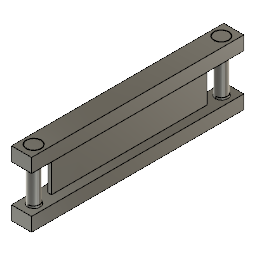
Treads v2 (Autodesk Fusion 360 design; units mm, degrees)
Autodesk Fusion 360 part; units mm, degrees
note: some values were not read from the file. Chosen so that the rebuilt part matches the saved one: which bodies a step acts on; which face or edge a step refers to.
sketch "Sketch1" plane through (0, 0, 0) normal (0, 0, 1) x (1, 0, 0)
  line L0 (0, 0) -> (11.5, 0)
  line L1 (11.5, 0) -> (11.5, 40)
  line L2 (11.5, 40) -> (0, 40)
  line L3 (0, 40) -> (0, 0)
  dimension "d1" = 11.5
  dimension "d2" = 40
  constraint horizontal L0
  constraint vertical L1
  constraint horizontal L2
  constraint vertical L3
  constraint coincident L0.start L3.end
  measures "d1" distance of L0.start L0.end
  measures "d2" distance of L0.start L2.end
extrude "Extrude1" add sketch "Sketch1" along normal blind 7.85 makes body 1
sketch "Sketch2" plane through (0, 0, 7.85) normal (0, 0, 1) x (-1, 0, 0)
  line L0 (0, -40) -> (0, 0)
  line L1 (0, 0) -> (-11.5, 0)
  line L2 (-11.5, 0) -> (-11.5, -40)
  line L3 (-11.5, -40) -> (0, -40)
  circle A0 centre (-5.6811, -7) radius 3.5
  circle A1 centre (-5.6811, -7) radius 3.25
  circle A2 centre (-5.6811, -7) radius 4
  circle A3 centre (-5.6811, -7) radius 4.25
  circle A4 centre (-5.6811, -33) radius 3.25
  circle A5 centre (-5.6811, -33) radius 3.5
  circle A6 centre (-5.6811, -33) radius 4
  circle A7 centre (-5.6811, -33) radius 4.25
  dimension "d5" = 7
  dimension "d6" = 6.5
  dimension "d7" = 8
  dimension "d12" = 8.5
  dimension "d17" = 7
  dimension "d18" = 7
  dimension "d19" = 6.5
  dimension "d20" = 8
  dimension "d21" = 8.5
  dimension "d22" = 7
  constraint concentric A0 A1
  constraint concentric A0 A2
  constraint concentric A1 A3
  constraint concentric A4 A5
  constraint concentric A5 A6
  constraint concentric A4 A7
  measures "d5" diameter of A0
  measures "d6" diameter of A1
  measures "d7" diameter of A2
  measures "d12" diameter of A3
  measures "d17" distance of L1 A0.centre
  measures "d18" diameter of A5
  measures "d19" diameter of A4
  measures "d20" diameter of A6
  measures "d21" diameter of A7
  measures "d22" distance of L3 A4.centre
extrude "Extrude2" cut sketch "Sketch2" against normal blind 2 contours A2 | A3 | A6 | A7 bodies 1
extrude "Extrude3" cut sketch "Sketch2" against normal blind 14 contours A0 | A5 bodies 1 makes body 2 at (5.8142, 1.1699, 0) makes body 3 at (2.4351, 33.162, 5.2333)
extrude "Extrude4" add sketch "Sketch2" along normal blind 1 contours A0 | A1 | A2 | A4 | A5 | A6 bodies 1 3
move_body "Move1" bodies 3 1 to x (1, 0, 0) y (0, 1, 0) z (0, 0, 1) at (0, 0, 0)
move_body "Move3" bodies 3 1 2 to x (-1, 0, 0) y (0, 1, 0) z (0, 0, -1) at (11.5, 0, 20)
copy_body "CopyPasteBodies1" bodies 2 1 3 makes body 4 makes body 5 makes body 6
move_body "Move4" bodies 4 5 6 to x (1, 0, 0) y (0, 1, 0) z (0, 0, 1) at (0, 0, 25)
move_body "Move5" bodies 6 5 4 to x (-1, 0, 0) y (0, 1, 0) z (0, 0, -1) at (11.5, 0, 86)
extrude "Extrude6" add 2 faces at (6.835, 5.7355, 41) (5.762, 31.968, 41) along direction (0, 0, -1) blind 27 on bodies 5 6 bodies 5 3 1 6
sketch "Sketch3" plane through (0, 0, 20) normal (0, 0, 1) x (-1, 0, 0)
  circle A0 centre (-5.8189, -7) radius 3.5
  circle A1 centre (-5.8189, -33) radius 3.5
  line L0 (-11.5, 0) -> (-11.5, -40)
  line L1 (-11.5, -40) -> (0, -40)
  line L2 (0, -40) -> (0, 0)
  line L3 (0, 0) -> (-11.5, 0)
  line L4 (-4.4693, -24.2011) -> (-6.5364, -24.2011)
  line L5 (-6.5364, -24.2011) -> (-6.5364, -16.2011)
  line L6 (-6.5364, -16.2011) -> (-4.4693, -16.2011)
  line L7 (-4.4693, -16.2011) -> (-4.4693, -24.2011)
  constraint horizontal L4
  constraint vertical L5
  constraint horizontal L6
  constraint vertical L7
extrude "Extrude7" add sketch "Sketch3" along normal blind 24 contours L4 L5 L6 L7 bodies 4 2
ref_plane "WorkPlane1" through (0, 0, 29) normal (0, 0, 1) x (1, 0, 0)
split "Split1" by plane through (0, 0, 29) normal (0, 0, 1) bodies 3 5 makes body 8 at (2.4351, 7.162, 35.6167) makes body 7 at (2.4351, 33.162, 35.6167)
extrude "Extrude8" cut 2 faces at (6.4361, 6.6807, 29) (7.213, 33.5625, 29) along direction (0, 0, -1) blind 2 on bodies 3 5 bodies 3 5
move_body "Move6" bodies 7 8 to x (1, 0, 0) y (0, 1, 0) z (0, 0, 1) at (0, 0, -1)
move_body "Move7" bodies 5 3 to x (1, 0, 0) y (0, 1, 0) z (0, 0, 1) at (0, 0, 1)
combine "Combine1" operation add target body 3 tool bodies 7
combine "Combine2" operation add target body 5 tool bodies 8
move_body "Move8" bodies 5 4 3 to x (1, 0, 0) y (0, 1, 0) z (0, 0, 1) at (0, 0, -12)
ref_plane "WorkPlane2" through (0, 20, 0) normal (0, 1, 0) x (0, 0, 1)
split "Split2" by plane through (0, 20, 0) normal (0, 1, 0) bodies 5 3 4 makes body 9 at (8.807, 24.9402, 8)
move_body "Move9" bodies 9 3 to x (1, 0, 0) y (0, 1, 0) z (0, 0, 1) at (0, 50, 0)
move_body "Move10" bodies 9 3 to x (1, 0, 0) y (0, 1, 0) z (0, 0, 1) at (0, 60, 0)
extrude "Extrude9" add 1 faces at (6.0121, 20, 34.2333) along direction (0, 1, 0) blind 80 on bodies 4 bodies 4
move_body "Move11" bodies 3 9 to x (1, 0, 0) y (0, 1, 0) z (0, 0, 1) at (0, -30, 0)
combine "Combine3" operation add target body 4 tool bodies 9
named bodies: "full body", "full body (1)"
